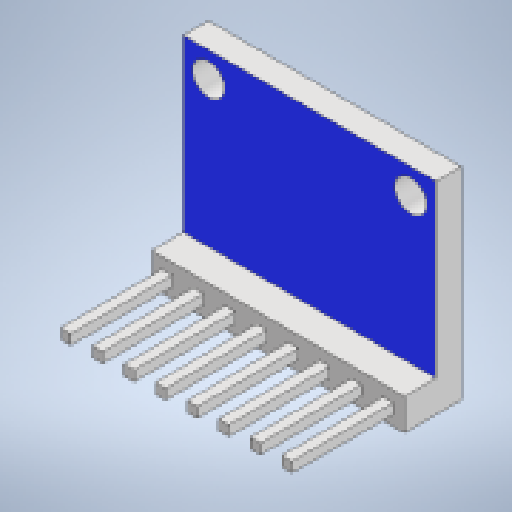
# Autodesk Inventor part: gyro
Saved by Autodesk Inventor 2024 (Build 280153000, 153)
## iProperties
Created: 2024-03-16
Part Number: gyro
Material: Générique
Document SubType Name: Modeling
Designer: phaly
Density: 1 g/cm^3
Appearance: Par défaut
Author: phaly
Autodesk Inventor part; units mm, degrees
ref_plane "YZ Plane" through (0, 0, 0) normal (1, 0, 0) x (0, 1, 0)
ref_plane "XZ Plane" through (0, 0, 0) normal (0, 1, 0) x (-1, 0, 0)
ref_plane "XY Plane" through (0, 0, 0) normal (0, 0, 1) x (1, 0, 0)
sketch "Esquisse1" plane through (0, 0, 0) normal (0, 0, 1) x (1, 0, 0)
  line L0 (0, 16) -> (20, 16)
  line L1 (20, 16) -> (20, 0)
  line L2 (20, 0) -> (0, 0)
  line L3 (0, 0) -> (0, 16)
  line L4 (-4.5575, 0) -> (27.3449, 0) projected
  line L5 (0, -3.2) -> (0, 19.2) projected
  point P0 (0, 0)
  dimension "d0" = 20
  dimension "d1" = 16
  constraints: 8 end point, 2 collinear, 2 parallel, 1 horizontal, 1 perpendicular
  measures "d0" distance of L0.start L0.end
  measures "d1" distance between parallel lines of L2 L0
extrude "Extrusion1" add sketch "Esquisse1" along normal blind 2
sketch "Esquisse2" plane through (0, 0, 2) normal (0, 0, 1) x (1, 0, 0)
  line L0 (20, 0) -> (20, 16) projected
  line L1 (20, 16) -> (0, 16) projected
  line L2 (0, 16) -> (0, 0) projected
  point P0 (2, 14)
  point P1 (18, 14)
  dimension "d11" = 2
  dimension "d12" = 2
  dimension "d13" = 2
  dimension "d14" = 2
  measures "d11" distance from line of L0 point (18, 14)
  measures "d12" distance from line of point (18, 14) L1
  measures "d13" distance from line of L1 point (2, 14)
  measures "d14" distance from line of L2 point (2, 14)
hole "Perçage1" at (2, 14, 2) at (18, 14, 2) direction (0, 0, -1) diameter 2.5 end through all
sketch "Esquisse3" plane through (0, 0, 2) normal (0, 0, 1) x (1, 0, 0)
  line L0 (0, 2.5) -> (2.5, 2.5)
  line L1 (2.5, 2.5) -> (2.5, 0)
  line L2 (2.5, 0) -> (0, 0)
  line L3 (0, 0) -> (0, 2.5)
  line L4 (-4.5575, 0) -> (27.3449, 0) projected
  line L5 (2.5, 2.5) -> (5, 2.5)
  line L6 (5, 2.5) -> (5, 0)
  line L7 (5, 0) -> (2.5, 0)
  line L8 (2.5, 0) -> (2.5, 2.5)
  line L9 (5, 2.5) -> (7.5, 2.5)
  line L10 (7.5, 2.5) -> (7.5, 0)
  line L11 (7.5, 0) -> (5, 0)
  line L12 (5, 0) -> (5, 2.5)
  line L13 (7.5, 2.5) -> (10, 2.5)
  line L14 (10, 2.5) -> (10, 0)
  line L15 (10, 0) -> (7.5, 0)
  line L16 (7.5, 0) -> (7.5, 2.5)
  line L17 (10, 2.5) -> (12.5, 2.5)
  line L18 (12.5, 2.5) -> (12.5, 0)
  line L19 (12.5, 0) -> (10, 0)
  line L20 (10, 0) -> (10, 2.5)
  line L21 (12.5, 2.5) -> (15, 2.5)
  line L22 (15, 2.5) -> (15, 0)
  line L23 (15, 0) -> (12.5, 0)
  line L24 (12.5, 0) -> (12.5, 2.5)
  line L25 (15, 2.5) -> (17.5, 2.5)
  line L26 (17.5, 2.5) -> (17.5, 0)
  line L27 (17.5, 0) -> (15, 0)
  line L28 (15, 0) -> (15, 2.5)
  line L29 (17.5, 2.5) -> (20, 2.5)
  line L30 (20, 2.5) -> (20, 0)
  line L31 (20, 0) -> (17.5, 0)
  line L32 (17.5, 0) -> (17.5, 2.5)
  line L33 (0, 16) -> (0, 0) projected
  line L34 (0, 0) -> (20, 0) projected
  point P0 (2.5, 0)
  point P1 (20, 0)
  dimension "d15" = 2.5
  dimension "d16" = 2.5
  dimension "d19" = 2.5
  constraints: 64 end point, 2 collinear, 2 horizontal, 2 parallel, 1 perpendicular, 56 other
  measures "d15" distance of L0.start L0.end
  measures "d16" distance of L2.end L0.start
  measures "d19" distance of L0.start L5.start
extrude "Extrusion2" add sketch "Esquisse3" along normal blind 2.5
sketch "Esquisse4" plane through (0, 0, 4.5) normal (0, 0, 1) x (1, 0, 0)
  line L0 (0.8, 1.6) -> (1.6, 1.6)
  line L1 (1.6, 1.6) -> (1.6, 0.8)
  line L2 (1.6, 0.8) -> (0.8, 0.8)
  line L3 (0.8, 0.8) -> (0.8, 1.6)
  line L4 (0, 0) -> (20, 0) projected
  line L5 (0, 2.5) -> (0, 0) projected
  line L6 (3.3, 1.6) -> (4.1, 1.6)
  line L7 (4.1, 1.6) -> (4.1, 0.8)
  line L8 (4.1, 0.8) -> (3.3, 0.8)
  line L9 (3.3, 0.8) -> (3.3, 1.6)
  line L10 (5.8, 1.6) -> (6.6, 1.6)
  line L11 (6.6, 1.6) -> (6.6, 0.8)
  line L12 (6.6, 0.8) -> (5.8, 0.8)
  line L13 (5.8, 0.8) -> (5.8, 1.6)
  line L14 (8.3, 1.6) -> (9.1, 1.6)
  line L15 (9.1, 1.6) -> (9.1, 0.8)
  line L16 (9.1, 0.8) -> (8.3, 0.8)
  line L17 (8.3, 0.8) -> (8.3, 1.6)
  line L18 (10.8, 1.6) -> (11.6, 1.6)
  line L19 (11.6, 1.6) -> (11.6, 0.8)
  line L20 (11.6, 0.8) -> (10.8, 0.8)
  line L21 (10.8, 0.8) -> (10.8, 1.6)
  line L22 (13.3, 1.6) -> (14.1, 1.6)
  line L23 (14.1, 1.6) -> (14.1, 0.8)
  line L24 (14.1, 0.8) -> (13.3, 0.8)
  line L25 (13.3, 0.8) -> (13.3, 1.6)
  line L26 (15.8, 1.6) -> (16.6, 1.6)
  line L27 (16.6, 1.6) -> (16.6, 0.8)
  line L28 (16.6, 0.8) -> (15.8, 0.8)
  line L29 (15.8, 0.8) -> (15.8, 1.6)
  line L30 (18.3, 1.6) -> (19.1, 1.6)
  line L31 (19.1, 1.6) -> (19.1, 0.8)
  line L32 (19.1, 0.8) -> (18.3, 0.8)
  line L33 (18.3, 0.8) -> (18.3, 1.6)
  point P0 (0, 1.25)
  dimension "d26" = 0.8
  dimension "d27" = 0.8
  dimension "d28" = 0.8
  dimension "d29" = 0.8
  dimension "d32" = 2.5
  constraints: 64 end point, 2 horizontal, 2 parallel, 1 midpoint, 1 perpendicular, 56 other
  measures "d26" distance of L0.start L0.end
  measures "d27" distance of L2.end L0.start
  measures "d28" distance between parallel lines of L4 L2
  measures "d29" distance from line of point (0, 1.25) L3
  measures "d32" distance of L0.start L6.start
extrude "Extrusion3" add sketch "Esquisse4" along normal blind 8
equation "\"d13\" = d12"
equation "\"d14\" = d11"
equation "\"d16\" = d15"
equation "\"d27\" = d26"
equation "\"d29\" = d28"
